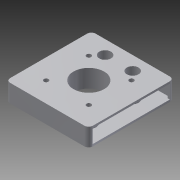
# Autodesk Inventor part: NEMA17-mount-plastic
Saved by Autodesk Inventor 2015 (Build 190159000, 159)
## iProperties
Created: 2012-03-11
Part Number: NEMA17-mount-plastic
Material: Generic
Document SubType Name: Modeling
Designer: Michael Green
Density: 1 g/cm^3
Appearance: Default
Author: Michael Green
Autodesk Inventor part; units mm, degrees
ref_plane "YZ Plane" through (0, 0, 0) normal (1, 0, 0) x (0, 1, 0)
ref_plane "XZ Plane" through (0, 0, 0) normal (0, 1, 0) x (-1, 0, 0)
ref_plane "XY Plane" through (0, 0, 0) normal (0, 0, 1) x (1, 0, 0)
sketch "base-drawing" plane through (0, 0, 0) normal (0, 0, 1) x (1, 0, 0)
  circle A0 centre (30, 30.15) radius 11.1
  circle A1 centre (20, 52) radius 2.65
  circle A2 centre (40, 52) radius 2.65
  line L0 (0, 0) -> (60, 0)
  line L1 (60, 0) -> (60, 62)
  line L2 (0, 62) -> (0, 0)
  line L3 (0, 62) -> (60, 62)
  circle A3 centre (45.5, 14.65) radius 1.7
  circle A4 centre (45.5, 45.65) radius 1.7
  circle A5 centre (14.5, 45.65) radius 1.7
  circle A6 centre (14.5, 14.65) radius 1.7
  dimension "d17" = 22.2
  dimension "d82" = 3.4
  dimension "d83" = 15.5
  dimension "d84" = 15.5
  dimension "d85" = 5.3
  dimension "d88" = 360
  dimension "d110" = 62
  dimension "d111" = 60
  constraints: 8 end point, 7 centre point, 2 perpendicular, 1 equal radius, 1 horizontal, 1 parallel, 9 other
  measures "d17" diameter of A0
  measures "d82" diameter of A3
  measures "d83" horizontal distance of A3.centre A0.centre
  measures "d84" horizontal distance of A0.centre A3.centre
  measures "d85" diameter of A2
  measures "d110" distance between parallel lines of L0 L3
  measures "d111" distance between parallel lines of L1 L2
extrude "Extrusion3" add sketch "base-drawing" along normal blind 13
sketch "Sketch10" plane through (0, 0, 13) normal (0, 0, 1) x (1, 0, 0)
  circle A0 centre (40, 52) radius 2.65 projected
  circle A1 centre (20, 52) radius 2.65 projected
  constraints: 2 coincident
hole "Hole7" at (20, 52, 13) at (40, 52, 13) direction (0, 0, -1) diameter 8.55 depth 8
sketch "Sketch12" plane through (0, 0, 0) normal (0, 0, -1) x (-1, 0, 0)
  circle A0 centre (-14.5, 14.65) radius 1.7 projected
  circle A1 centre (-14.5, 45.65) radius 1.7 projected
  circle A2 centre (-45.5, 45.65) radius 1.7 projected
  circle A3 centre (-45.5, 14.65) radius 1.7 projected
  constraints: 4 coincident
hole "Hole8" at (45.5, 45.65, 0) at (14.5, 45.65, 0) at (14.5, 14.65, 0) at (45.5, 14.65, 0) direction (0, 0, 1) diameter 7.3 depth 6.4
fillet "Fillet3" radius 3 4 edges at (60, 62, 6.5) (0, 62, 6.5) (0, 0, 6.5) (60, 0, 6.5)
shell "Shell5" thickness 1.5 removed faces 2 at (60, 21.6667, 4.3333) at (0, 40.3333, 4.3333)
body "Solid3"
